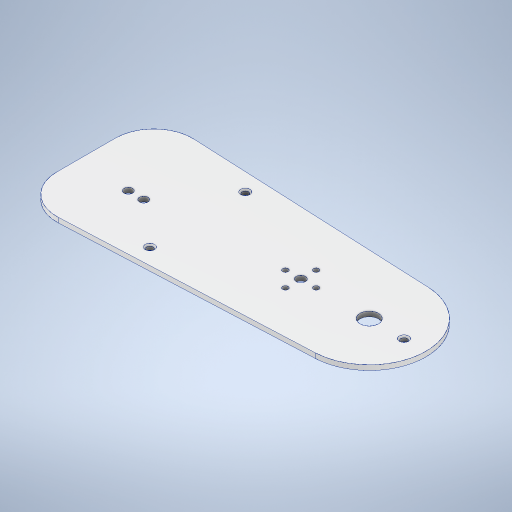
# Autodesk Inventor part: Wrist Side Brase
Saved by Autodesk Inventor 2023 (Build 270158030, 158C)
## iProperties
Created: 2022-09-21
Part Number: Wrist Side Brase
Material: Aluminum 6061
Document SubType Name: Modeling
Designer: caden
Density: 2.7 g/cm^3
Appearance: Aluminum - Flat
Mass: 158.416 g
Surface Area: 396.255 cm^2
Volume: 58.6727 cm^3
Author: caden
Autodesk Inventor part; units mm, degrees
ref_plane "YZ Plane" through (0, 0, 0) normal (1, 0, 0) x (0, 1, 0)
ref_plane "XZ Plane" through (0, 0, 0) normal (0, 1, 0) x (-1, 0, 0)
ref_plane "XY Plane" through (0, 0, 0) normal (0, 0, 1) x (1, 0, 0)
sketch "Sketch1" plane through (0, 0, 0) normal (0, 1, 0) x (-1, 0, 0)
  arc A0 (-1.6679, 36.7922) -> (-1.6679, -36.7922) centre (0, 0) ccw
  arc A1 (157.8679, -44.0244) -> (184, -19.05) centre (159, -19.05) ccw
  arc A2 (184, 19.05) -> (157.8679, 44.0244) centre (159, 19.05) ccw
  line L0 (157.8679, -44.0244) -> (-1.6679, -36.7922)
  line L1 (157.8679, 44.0244) -> (-1.6679, 36.7922)
  line L2 (184, -19.05) -> (184, 19.05)
  line L3 (0, 0) -> (1115.1702, 0)
  dimension "d0" = 50
  dimension "d1" = 159
  dimension "d2" = 38.1
  dimension "d3" = 36.83
  constraints: 8 end point, 6 point on circle, 6 tangent, 3 centre point, 1 coincident, 1 equal radius, 1 horizontal, 1 symmetric about line, 1 vertical
  measures "d0" diameter of A1
  measures "d1" horizontal distance of point (0, 0) A1.centre
  measures "d2" distance of A1.centre A2.centre
  measures "d3" radius of A0
extrude "Main" add sketch "Sketch1" along normal blind 3.175
sketch "Sketch2" plane through (0, 3.175, 0) normal (0, 1, 0) x (1, 0, 0)
  circle A0 centre (0, 0) radius 6
  circle A1 centre (-44.4754, 0) radius 3
  arc A2 (-184, -19.05) -> (-157.8679, -44.0244) centre (-159, -19.05) ccw projected
  arc A3 (-157.8679, 44.0244) -> (-184, 19.05) centre (-159, 19.05) ccw projected
  line L0 (0, 0) -> (-245.2379, 0)
  dimension "d6" = 6
  dimension "d40" = 12
  dimension "d41" = 44.4754
  constraints: 2 centre point, 2 end point, 1 coincident, 1 horizontal, 1 point on line
  measures "d6" diameter of A1
  measures "d40" diameter of A0
  measures "d41" distance of point (0, 0) A1.centre
extrude "Axis Holes" cut sketch "Sketch2" against normal through all
sketch "Sketch5" plane through (0, 3.175, 0) normal (0, 1, 0) x (1, 0, 0)
  line L0 (-133.2, -6.35) -> (-133.2, 29.1375) construction
  line L1 (-184, 19.05) -> (-184, -19.05) construction
  circle A0 centre (-140.2, -6.35) radius 2.75
  circle A1 centre (-150.2, -6.35) radius 2.75
  point P0 (0, 0)
  dimension "d43" = 50.8
  dimension "d44" = 7
  dimension "d45" = 10
  dimension "d46" = 5.5
  constraints: 2 centre point, 2 end point, 1 equal radius, 1 vertical
  measures "d43" distance between parallel lines of L0 L1
  measures "d44" distance from line of L0 A0.centre
  measures "d45" distance of A1.centre A0.centre
  measures "d46" diameter of A1
extrude "Extrusion6" cut sketch "Sketch5" against normal through all
sketch "Sketch7" plane through (0, 3.175, 0) normal (0, 1, 0) x (1, 0, 0)
  circle A0 centre (-44.4754, 0) radius 3 construction
  circle A1 centre (-44.4754, 0) radius 10 construction
  circle A2 centre (-44.4754, 10) radius 1.75
  circle A3 centre (-54.4754, 0) radius 1.75
  circle A4 centre (-44.4754, -10) radius 1.75
  circle A5 centre (-34.4754, 0) radius 1.75
  point P0 (0, 0)
  dimension "d63" = 20
  dimension "d58" = 3.5
  dimension "d61" = 360
  constraints: 4 centre point, 1 coincident, 1 vertical alignment, 11 other
  measures "d58" diameter of A2
extrude "Extrusion8" cut sketch "Sketch7" against normal blind 10
sketch "Sketch9" plane through (0, 3.175, 0) normal (0, 1, 0) x (1, 0, 0)
  circle A0 centre (-44.4754, 0) radius 3 projected
  point P0 (0, 0)
  point P1 (-12.3688, -17.5481)
  point P2 (-111.5344, -31)
  point P3 (-111.5344, 31)
  point P4 (22.5836, 0)
  dimension "d73" = 67.059
  dimension "d74" = 67.059
  dimension "d75" = 31
  dimension "d76" = 31
  constraints: 1 vertical alignment
  measures "d73" horizontal distance of A0.centre point (-111.534, 31)
  measures "d74" distance of A0.centre point (22.584, 0)
  measures "d75" vertical distance of A0.centre point (-111.534, -31)
  measures "d76" vertical distance of A0.centre point (-111.534, 31)
hole "Hole1" at (-111.5344, 3.175, 31) at (-111.5344, 3.175, -31) at (22.5836, 3.175, 0) direction (0, -1, 0) diameter 4.134 end through all countersink diameter 6 countersink angle 90 thread size "M5x0.8" class "6H" standard "ISO Metric profile"
body "Solid1"
